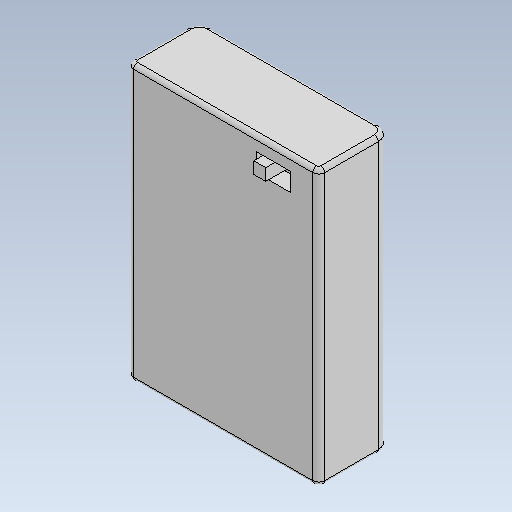
# Autodesk Inventor part: batt_box
Saved by Autodesk Inventor 2026.1 (Build 301233020, 233B)
## iProperties
Created: 2026-08-13
Part Number: batt_box
Material: 一般
Document SubType Name: Modeling
Designer: ug_nd
Density: 1 g/cm^3
Appearance: 既定
Author: ug_nd
Autodesk Inventor part; units mm, degrees
ref_plane "YZ Plane" through (0, 0, 0) normal (1, 0, 0) x (0, 1, 0)
ref_plane "XZ Plane" through (0, 0, 0) normal (0, 1, 0) x (-1, 0, 0)
ref_plane "XY Plane" through (0, 0, 0) normal (0, 0, 1) x (1, 0, 0)
sketch "スケッチ1" plane through (0, 0, 0) normal (0, 0, 1) x (1, 0, 0)
  line L0 (-24, -34.5) -> (24, -34.5)
  line L1 (24, -34.5) -> (24, 34.5)
  line L2 (24, 34.5) -> (-24, 34.5)
  line L3 (-24, 34.5) -> (-24, -34.5)
  line L4 (-24, -34.5) -> (24, 34.5) construction
  line L5 (24, -34.5) -> (-24, 34.5) construction
  point P0 (0, 0)
  dimension "d0" = 48
  dimension "d1" = 69
  constraints: 12 end point, 2 midpoint, 2 parallel, 1 horizontal, 1 perpendicular
  measures "d0" distance of L1.end L2.end
  measures "d1" distance of L2.end L0.start
extrude "押し出し1" add sketch "スケッチ1" along normal mid plane 18
fillet "フィレット1" radius 3 2 edges at (24, 0, -9) (-24, 0, -9)
fillet "フィレット2" radius 1.5 2 edges at (24, 0, 9) (-24, 0, 9)
fillet "フィレット3" radius 1 16 edges at (-23.5607, 34.5, 8.5607) (-24, 34.5, 0.75) (-23.1213, 34.5, -8.1213) (0, 34.5, -9) (23.1213, 34.5, -8.1213) (24, 34.5, 0.75) (23.5607, 34.5, 8.5607) (0, 34.5, 9) (23.5607, -34.5, 8.5607) (24, -34.5, 0.75) (23.1213, -34.5, -8.1213) (0, -34.5, -9) (-23.1213, -34.5, -8.1213) (-24, -34.5, 0.75) (-23.5607, -34.5, 8.5607) (0, -34.5, 9)
sketch "スケッチ2" plane through (0, 0, 9) normal (0, 0, 1) x (1, 0, 0)
  line L0 (8.4, 26.4) -> (17, 26.4)
  line L1 (17, 26.4) -> (17, 31)
  line L2 (17, 31) -> (8.4, 31)
  line L3 (8.4, 31) -> (8.4, 26.4)
  line L4 (8.4, 26.4) -> (17, 31) construction
  line L5 (17, 26.4) -> (8.4, 31) construction
  line L6 (24, -33.5) -> (24, 33.5) construction
  line L7 (22.5, 34.5) -> (-22.5, 34.5) construction
  point P0 (0, 0)
  point P1 (12.7, 28.7)
  dimension "d7" = 7
  dimension "d8" = 3.5
  dimension "d9" = 4.6
  dimension "d10" = 8.6
  constraints: 12 end point, 2 midpoint, 2 parallel, 1 horizontal, 1 perpendicular
  measures "d7" distance between parallel lines of L6 L1
  measures "d8" distance between parallel lines of L7 L2
  measures "d9" distance of L0.end L1.end
  measures "d10" distance of L1.end L2.end
extrude "押し出し2" cut sketch "スケッチ2" against normal blind 4
sketch "スケッチ3" plane through (0, 0, 5) normal (0, 0, 1) x (1, 0, 0)
  line L0 (17, 31) -> (17, 26.4) construction
  line L1 (8.4, 31) -> (17, 31) construction
  line L2 (8.4, 26.4) -> (8.4, 31) construction
  line L3 (17, 26.4) -> (8.4, 26.4) construction
  line L4 (8.4, 28.7) -> (17, 28.7) construction
  line L5 (12.2, 27.2) -> (9.2, 27.2)
  line L6 (9.2, 27.2) -> (9.2, 30.2)
  line L7 (9.2, 30.2) -> (12.2, 30.2)
  line L8 (12.2, 30.2) -> (12.2, 27.2)
  line L9 (12.2, 27.2) -> (9.2, 30.2) construction
  line L10 (9.2, 27.2) -> (12.2, 30.2) construction
  point P0 (0, 0)
  point P1 (10.7, 28.7)
  dimension "d13" = 3
  dimension "d14" = 3
  dimension "d15" = 0.8
  constraints: 14 end point, 4 midpoint, 2 parallel, 1 horizontal, 1 perpendicular, 1 point on line
  measures "d13" distance of L6.end L7.end
  measures "d14" distance of L5.end L6.end
  measures "d15" distance between parallel lines of L2 L6
extrude "押し出し3" add sketch "スケッチ3" along normal blind 5.5
